# Autodesk Inventor part: 15A
Saved by Autodesk Inventor 2016 (Build 200138000, 138)
## iProperties
Created: 2016-04-08
Part Number: 15A
Material: Generic
Document SubType Name: Modeling
Designer: Paschalis
Density: 1 g/cm^3
Appearance: PAS_5X20, 15A
Author: Paschalis
Autodesk Inventor part; units mm, degrees
ref_plane "YZ Plane" through (0, 0, 0) normal (1, 0, 0) x (0, 1, 0)
ref_plane "XZ Plane" through (0, 0, 0) normal (0, 1, 0) x (-1, 0, 0)
ref_plane "XY Plane" through (0, 0, 0) normal (0, 0, 1) x (1, 0, 0)
sketch "PAS_5X20, 15A_63" plane through (0, 0, 0) normal (0, 0, 1) x (1, 0, 0)
  line L0 (-15.5575, 1.9685) -> (-7.4295, 1.9685)
  line L1 (-7.4295, 1.9685) -> (-7.4295, -1.905)
  line L2 (-7.4295, -1.905) -> (-15.5575, -1.905)
  line L3 (-15.5575, -1.905) -> (-15.5575, 1.9685)
  constraints: 8 end point
extrude "Extrusion1" add sketch "PAS_5X20, 15A_63" along normal blind 1
body "Solid1"
